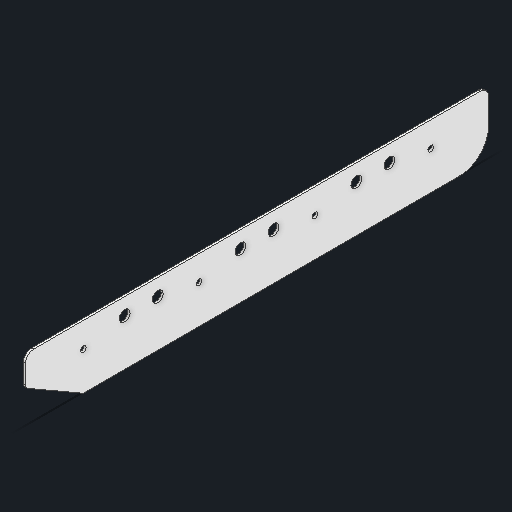
# Autodesk Inventor part: Skirt
Saved by Autodesk Inventor 2025.1 (Build 291241000, 241)
## iProperties
Created: 2024-12-17
Part Number: Skirt
Material: Acetal Resin, White
Document SubType Name: Modeling
Designer: Averey Ku
Density: 1.425 g/cm^3
Appearance: Smooth - White
Author: Averey Ku
Autodesk Inventor part; units mm, degrees
ref_plane "YZ Plane" through (0, 0, 0) normal (1, 0, 0) x (0, 1, 0)
ref_plane "XZ Plane" through (0, 0, 0) normal (0, 1, 0) x (-1, 0, 0)
ref_plane "XY Plane" through (0, 0, 0) normal (0, 0, 1) x (1, 0, 0)
sketch "main" plane through (0, 0, 0) normal (0, 0, 1) x (1, 0, 0)
  circle A0 centre (-6.8277, 139.0371) radius 2.1844
  circle A1 centre (-0.4777, 107.2871) radius 4.191
  line L0 (-8.7029, 183.4871) -> (6.7737, 183.4871)
  circle A2 centre (-6.8277, 50.1371) radius 2.1844
  circle A3 centre (-6.8277, -38.7629) radius 2.1844
  circle A4 centre (-6.8277, -127.6629) radius 2.1844
  circle A5 centre (-0.4777, 81.8871) radius 4.191
  circle A6 centre (-0.4777, 18.3871) radius 4.191
  line L1 (-36.1964, -149.8879) -> (-36.1964, 139.0371)
  circle A7 centre (-0.4777, -70.5129) radius 4.191
  circle A8 centre (-0.4777, -95.9129) radius 4.191
  line L2 (6.7053, -172.1129) -> (5.8723, -172.1129)
  line L3 (-13.9714, -172.1129) -> (6.7053, -172.1129)
  arc A9 (-36.1964, -149.8879) -> (-13.9714, -172.1129) centre (-13.9714, -149.8879) ccw
  circle A10 centre (-0.4777, -7.0129) radius 4.191
  line L4 (-11.4526, 181.8995) -> (-36.1964, 139.0371)
  arc A11 (-8.7029, 183.4871) -> (-11.4526, 181.8995) centre (-8.7029, 180.3121) ccw
  line L5 (-8.7029, 183.4871) -> (5.8723, 183.4871)
  line L6 (12.2223, 177.1371) -> (12.2223, -165.7629)
  arc A12 (12.2223, 177.1371) -> (5.8723, 183.4871) centre (5.8723, 177.1371) ccw
  arc A13 (5.8723, -172.1129) -> (12.2223, -165.7629) centre (5.8723, -165.7629) ccw
  point P0 (2.0753, 1.669)
  point P1 (-10.536, 183.4871)
  point P2 (5.8723, 139.0371)
  point P3 (12.2223, 183.4871)
  dimension "d4" = 8.382
  dimension "d5" = 8.382
  dimension "d6" = 8.382
  dimension "d7" = 8.382
  dimension "d8" = 8.382
  dimension "d9" = 8.382
  dimension "d10" = 12.7
  dimension "d11" = 0
  dimension "d12" = 88.9
  dimension "d13" = 88.9
  dimension "d14" = 88.9
  dimension "d15" = 29.3687
  dimension "d16" = 3.175
  dimension "d18" = 6.35
  dimension "d19" = 6.35
  dimension "d20" = 22.225
  measures "d4" diameter of A1
  measures "d5" diameter of A5
  measures "d6" diameter of A6
  measures "d7" diameter of A10
  measures "d8" diameter of A7
  measures "d9" diameter of A8
  measures "d10" distance of point (5.872, 139.037) A0.centre
  measures "d11" vertical distance of point (5.872, 139.037) A0.centre
  measures "d12" distance of A0.centre A2.centre
  measures "d13" distance of A3.centre A2.centre
  measures "d14" distance of A4.centre A3.centre
  measures "d15" distance from line of A0.centre L1
  measures "d16" radius of A11
  measures "d18" radius of A12
  measures "d19" radius of A13
  measures "d20" radius of A9
sketch "Sketch1" plane through (0, 0, 0) normal (1, 0, 0) x (0, 1, 0)
  circle A0 centre (0, 0) radius 2.1844
  circle A1 centre (6.35, -31.75) radius 4.191
  line L0 (-1.8752, 44.45) -> (13.6014, 44.45)
  circle A2 centre (0, -88.9) radius 2.1844
  circle A3 centre (0, -177.8) radius 2.1844
  circle A4 centre (0, -266.7) radius 2.1844
  circle A5 centre (6.35, -57.15) radius 4.191
  circle A6 centre (6.35, -120.65) radius 4.191
  line L1 (-29.3687, -288.925) -> (-29.3687, 0)
  circle A7 centre (6.35, -209.55) radius 4.191
  circle A8 centre (6.35, -234.95) radius 4.191
  line L2 (13.533, -311.15) -> (12.7, -311.15)
  line L3 (-7.1437, -311.15) -> (13.533, -311.15)
  arc A9 (-29.3687, -288.925) -> (-7.1437, -311.15) centre (-7.1437, -288.925) ccw
  circle A10 centre (6.35, -146.05) radius 4.191
  line L4 (-4.6249, 42.8624) -> (-29.3687, 0)
  arc A11 (-1.8752, 44.45) -> (-4.6249, 42.8624) centre (-1.8752, 41.275) ccw
  line L5 (-1.8752, 44.45) -> (12.7, 44.45)
  line L6 (19.05, 38.1) -> (19.05, -304.8)
  arc A12 (19.05, 38.1) -> (12.7, 44.45) centre (12.7, 38.1) ccw
  arc A13 (12.7, -311.15) -> (19.05, -304.8) centre (12.7, -304.8) ccw
  constraints: 1 other
extrude "Extrusion1" add sketch "Sketch1" along normal blind 1.5875
body "Solid1"
